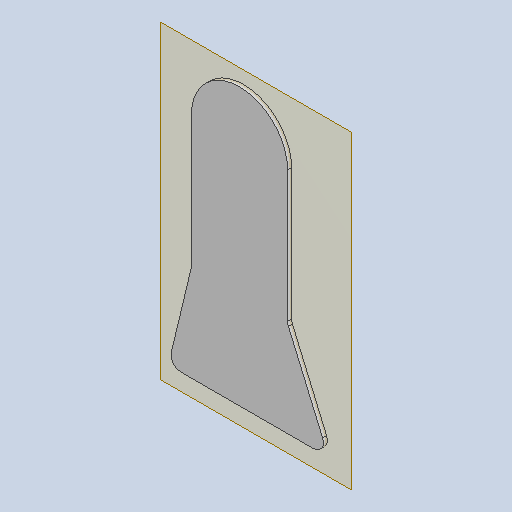
# Autodesk Inventor part: ребро
Saved by Autodesk Inventor 2023.1 (Build 271208000, 208)
## iProperties
Created: 2025-01-17
Part Number: ребро
Material: Типовые
Document SubType Name: Modeling
Designer: DELL
Density: 1 g/cm^3
Appearance: По умолчанию
Author: DELL
Autodesk Inventor part; units mm, degrees
ref_plane "YZ Plane" through (0, 0, 0) normal (1, 0, 0) x (0, 1, 0)
ref_plane "XZ Plane" through (0, 0, 0) normal (0, 1, 0) x (-1, 0, 0)
ref_plane "XY Plane" through (0, 0, 0) normal (0, 0, 1) x (1, 0, 0)
ref_plane "РабПлоскость1" through (0, 0, 0) normal (0, 0, 1) x (1, 0, 0)
sketch "Эскиз2" plane through (0, 0, 0) normal (0, 0, 1) x (1, 0, 0)
  line L0 (8.0047, 276) -> (12.0047, 276) construction
  line L1 (10.0047, 276) -> (10.0047, 0) construction
  line L2 (-37.9953, 228) -> (-37.9953, 97.1846)
  line L3 (58.0047, 97.1846) -> (58.0047, 228)
  arc A0 (58.0047, 228) -> (-37.9953, 228) centre (10.0047, 228) ccw
  line L4 (-48.3749, 0) -> (83.7223, 0)
  line L5 (92.9091, 13.9502) -> (58.818, 93.2344)
  line L6 (-38.2721, 94.8482) -> (-58.0982, 12.3363)
  arc A1 (58.0047, 97.1846) -> (58.818, 93.2344) centre (68.0047, 97.1846) ccw
  arc A2 (-38.2721, 94.8482) -> (-37.9953, 97.1846) centre (-47.9953, 97.1846) ccw
  arc A3 (83.7223, 0) -> (92.9091, 13.9502) centre (83.7223, 10) ccw
  arc A4 (-58.0982, 12.3363) -> (-48.3749, 0) centre (-48.3749, 10) ccw
  line L7 (-37.9953, 97.1846) -> (108, 97.1846) construction
  line L8 (110.0044, 0) -> (-61.0624, 0) projected
  point P0 (10.0047, 138)
  dimension "d11" = 10
  dimension "d12" = 10
  dimension "d13" = 10
  constraints: 16 end point, 11 point on circle, 10 tangent, 6 point on line, 5 centre point, 2 horizontal, 2 midpoint, 1 equal radius, 1 parallel, 1 perpendicular
  measures "d11" radius of A1
  measures "d12" radius of A2
  measures "d13" radius of A3
extrude "Выдавливание2" add sketch "Эскиз2" along normal mid plane 4
